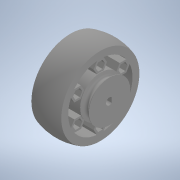
# Autodesk Inventor part: PulleyedWheelV1
Saved by Autodesk Inventor 2020 (Build 240168000, 168)
## iProperties
Created: 2023-12-21
Part Number: PulleyedWheelV1
Material: H TPU
Document SubType Name: Modeling
Designer: smz3rm
Density: 0.941117 g/cm^3
Appearance: Generic(1)
Mass: 15.4357 g
Surface Area: 101.181 cm^2
Volume: 16.4015 cm^3
d0: 3.000 mm
d1: 1.000 mm
d3: 34.000 mm
d4: 3.000 mm
d6: 18.000 mm
d7: 4.000 mm
d8: 0.00 deg
d9: 34.000 mm
d10: 1.600 mm
d11: 0.800 mm
d12: 6.000 ul
d16: 13.000 mm
d17: 0.00 deg
d20: 2.000 mm
d24: 1.000 mm
d26: 45.00 deg
Roundedness: 1.000 mm
d14: 360.00 deg
BaseThickness: 3.000 mm
TopThickness: 1.778 mm
SideThickness: 6.000 mm
BodyWidth: 130.000 mm
BodyLength: 150.000 mm
BodyHeight: 35.000 mm
DriveMotorHeight: 17.500 mm
WheelDia: 36.000 mm
WheelWidth: 13.000 mm
WheelGrooveWidth: 4.000 mm
WheelGrooveDia: 18.000 mm
WheelSlotWidth: 20.000 mm
WheelPulleyDia: 2.000 mm
WheeGuardlSlotWidth: 20.000 mm
Author: smz3rm
Autodesk Inventor part; units mm, degrees
ref_plane "YZ Plane" through (0, 0, 0) normal (1, 0, 0) x (0, 1, 0)
ref_plane "XZ Plane" through (0, 0, 0) normal (0, 1, 0) x (-1, 0, 0)
ref_plane "XY Plane" through (0, 0, 0) normal (0, 0, 1) x (1, 0, 0)
sketch "Sketch1" plane through (0, 0, 0) normal (1, 0, 0) x (0, 1, 0)
  circle A0 centre (0, 0) radius 1.5
  line L0 (-23.45, 0) -> (23.45, 0) projected
  line L1 (1.118, -1) -> (-1.118, -1)
  circle A1 centre (0, 0) radius 9
  circle A2 centre (0, 0) radius 17
  circle A3 centre (0, 0) radius 14
  dimension "d0" = 3
  dimension "d1" = 1
  dimension "d3" = 34
  dimension "d4" = 3
  dimension "d6" = 18
  constraints: 4 centre point, 4 coincident, 2 end point, 2 point on circle, 1 horizontal
  measures "d0" diameter of A0
  measures "d1" distance between parallel lines of L0 L1
  measures "d3" diameter of A2
  measures "d4" radial gap between concentric circles of A2 A3
  measures "d6" diameter of A1
extrude "Extrusion1" add sketch "Sketch1" along normal blind 4 contours L1 A0 | A0 L0 A1 | L0 A1 A0
sketch "Sketch3" plane through (0, 0, 0) normal (0, 0, 1) x (1, 0, 0)
  line L0 (0, 9) -> (4, 9) projected
  line L1 (-0.8, 0) -> (4.8, 0) projected
  circle A0 centre (1.3858, 8) radius 1
  line L2 (0.4001, 7.8312) -> (0.2, 9)
  line L3 (0, 9) -> (4, 9) projected
  line L4 (0, 10) -> (4, 10) projected
  line L5 (0, 9) -> (4, 9) projected
  line L6 (3.8, 9) -> (2.0929, 7.2929)
  line L7 (3.8, 9) -> (3.8, 9)
  line L8 (3.8, 9) -> (4, 9)
  line L9 (4, -9) -> (4, 9) projected
  line L10 (4, 9) -> (4, 9)
  line L11 (0, -9) -> (0, 9) projected
  line L12 (0.2, 9) -> (0, 9)
  point P0 (0, 0)
  point P1 (1.3858, 9)
  point P2 (3.8, 9)
  dimension "d20" = 2
  dimension "d26" = 45
  dimension "d28" = 0.2
  constraints: 12 end point, 3 perpendicular, 3 tangent, 2 collinear, 2 point on circle, 2 point on line, 1 centre point, 1 vertical, 3 other
  measures "d20" diameter of A0
  measures "d26" angle of L0 L6
  measures "d28" distance of L0.end L6.start
revolve "Revolution1" cut sketch "Sketch3" angle 360 about axis through (-10, 0, 0) along (-1, 0, 0) contours L0 A0 L2 | L0 L6 A0 | A0
sketch "Sketch2" plane through (0, 0, 0) normal (-1, 0, 0) x (0, 0, 1)
  circle A0 centre (0, 0) radius 17
  circle A1 centre (0, 0) radius 15.4
  circle A2 centre (0, 0) radius 9 projected
  line L0 (-1, 1.118) -> (-1, -1.118) projected
  arc A3 (-1, -1.118) -> (-1, 1.118) centre (0, 0) ccw projected
  line L1 (1.8714, 15.2859) -> (3.7427, 12.0446)
  line L2 (3.7427, 12.0446) -> (1.8714, 8.8033)
  line L3 (1.8714, 8.8033) -> (-1.8714, 8.8033)
  line L4 (-1.8714, 8.8033) -> (-3.7427, 12.0446)
  line L5 (-3.7427, 12.0446) -> (-1.8714, 15.2859)
  line L6 (-1.8714, 15.2859) -> (1.8714, 15.2859)
  line L7 (0, -23.45) -> (0, 23.45) projected
  line L8 (-1.4095, 14.4859) -> (-2.819, 12.0446)
  line L9 (-2.819, 12.0446) -> (-1.4095, 9.6033)
  line L10 (-1.4095, 9.6033) -> (1.4095, 9.6033)
  line L11 (1.4095, 9.6033) -> (2.819, 12.0446)
  line L12 (2.819, 12.0446) -> (1.4095, 14.4859)
  line L13 (1.4095, 14.4859) -> (-1.4095, 14.4859)
  line L14 (-12.3023, 2.781) -> (-14.1736, 6.0223)
  line L15 (-8.5596, 2.781) -> (-12.3023, 2.781)
  line L16 (-6.6882, 6.0223) -> (-8.5596, 2.781)
  line L17 (-14.1736, 6.0223) -> (-12.3023, 9.2636)
  line L18 (-12.3023, 9.2636) -> (-8.5596, 9.2636)
  line L19 (-8.5596, 9.2636) -> (-6.6882, 6.0223)
  line L20 (-11.8404, 8.4636) -> (-13.2499, 6.0223)
  line L21 (-13.2499, 6.0223) -> (-11.8404, 3.581)
  line L22 (-11.8404, 3.581) -> (-9.0214, 3.581)
  line L23 (-9.0214, 3.581) -> (-7.612, 6.0223)
  line L24 (-7.612, 6.0223) -> (-9.0214, 8.4636)
  line L25 (-9.0214, 8.4636) -> (-11.8404, 8.4636)
  line L26 (-8.5596, -9.2636) -> (-12.3023, -9.2636)
  line L27 (-6.6882, -6.0223) -> (-8.5596, -9.2636)
  line L28 (-8.5596, -2.781) -> (-6.6882, -6.0223)
  line L29 (-12.3023, -9.2636) -> (-14.1736, -6.0223)
  line L30 (-14.1736, -6.0223) -> (-12.3023, -2.781)
  line L31 (-12.3023, -2.781) -> (-8.5596, -2.781)
  line L32 (-13.2499, -6.0223) -> (-11.8404, -8.4636)
  line L33 (-11.8404, -8.4636) -> (-9.0214, -8.4636)
  line L34 (-9.0214, -8.4636) -> (-7.612, -6.0223)
  line L35 (-7.612, -6.0223) -> (-9.0214, -3.581)
  line L36 (-9.0214, -3.581) -> (-11.8404, -3.581)
  line L37 (-11.8404, -3.581) -> (-13.2499, -6.0223)
  line L38 (3.7427, -12.0446) -> (1.8714, -15.2859)
  line L39 (1.8714, -8.8033) -> (3.7427, -12.0446)
  line L40 (-1.8714, -8.8033) -> (1.8714, -8.8033)
  line L41 (1.8714, -15.2859) -> (-1.8714, -15.2859)
  line L42 (-1.8714, -15.2859) -> (-3.7427, -12.0446)
  line L43 (-3.7427, -12.0446) -> (-1.8714, -8.8033)
  line L44 (-1.4095, -14.4859) -> (1.4095, -14.4859)
  line L45 (1.4095, -14.4859) -> (2.819, -12.0446)
  line L46 (2.819, -12.0446) -> (1.4095, -9.6033)
  line L47 (1.4095, -9.6033) -> (-1.4095, -9.6033)
  line L48 (-1.4095, -9.6033) -> (-2.819, -12.0446)
  line L49 (-2.819, -12.0446) -> (-1.4095, -14.4859)
  line L50 (12.3023, -2.781) -> (14.1736, -6.0223)
  line L51 (8.5596, -2.781) -> (12.3023, -2.781)
  line L52 (6.6882, -6.0223) -> (8.5596, -2.781)
  line L53 (14.1736, -6.0223) -> (12.3023, -9.2636)
  line L54 (12.3023, -9.2636) -> (8.5596, -9.2636)
  line L55 (8.5596, -9.2636) -> (6.6882, -6.0223)
  line L56 (11.8404, -8.4636) -> (13.2499, -6.0223)
  line L57 (13.2499, -6.0223) -> (11.8404, -3.581)
  line L58 (11.8404, -3.581) -> (9.0214, -3.581)
  line L59 (9.0214, -3.581) -> (7.612, -6.0223)
  line L60 (7.612, -6.0223) -> (9.0214, -8.4636)
  line L61 (9.0214, -8.4636) -> (11.8404, -8.4636)
  line L62 (8.5596, 9.2636) -> (12.3023, 9.2636)
  line L63 (6.6882, 6.0223) -> (8.5596, 9.2636)
  line L64 (8.5596, 2.781) -> (6.6882, 6.0223)
  line L65 (12.3023, 9.2636) -> (14.1736, 6.0223)
  line L66 (14.1736, 6.0223) -> (12.3023, 2.781)
  line L67 (12.3023, 2.781) -> (8.5596, 2.781)
  line L68 (13.2499, 6.0223) -> (11.8404, 8.4636)
  line L69 (11.8404, 8.4636) -> (9.0214, 8.4636)
  line L70 (9.0214, 8.4636) -> (7.612, 6.0223)
  line L71 (7.612, 6.0223) -> (9.0214, 3.581)
  line L72 (9.0214, 3.581) -> (11.8404, 3.581)
  line L73 (11.8404, 3.581) -> (13.2499, 6.0223)
  point P0 (0, 12.0446)
  point P1 (-1.8714, -15.2859)
  point P2 (-12.3023, -9.2636)
  point P3 (-6.6882, -6.0223)
  point P4 (-1.8714, -8.8033)
  point P5 (-6.6882, 6.0223)
  point P6 (-12.3023, 9.2636)
  point P7 (12.3023, 9.2636)
  point P8 (6.6882, 6.0223)
  point P9 (1.8714, 8.8033)
  point P10 (14.1736, -6.0223)
  point P11 (8.5596, -2.781)
  point P12 (8.5596, 2.781)
  point P13 (14.1736, 6.0223)
  point P14 (1.8714, -15.2859)
  point P15 (1.8714, -8.8033)
  point P16 (12.3023, -9.2636)
  point P17 (-14.1736, 6.0223)
  point P18 (-8.5596, 2.781)
  point P19 (-8.5596, -2.781)
  point P20 (-14.1736, -6.0223)
  dimension "d9" = 34
  dimension "d10" = 1.6
  dimension "d11" = 0.8
  dimension "d14" = 360
  constraints: 144 end point, 2 centre point, 2 coincident, 2 point on circle, 1 point on line, 165 other
  measures "d9" diameter of A0
  measures "d10" radial gap between concentric circles of A0 A1
  measures "d11" distance between parallel lines of L5 L8
extrude "Extrusion2" add sketch "Sketch2" along normal blind 13 contours A0 L7 A1 | L7 A1 A0 | L7 L6 A1 | A1 L6 L7 | L7 L41 A1 | A1 L41 L7 | L1 L2 A2 L7 L10 L11 L12 L13 L6 | L6 L7 L13 L8 L9 L10 A2 L4 L5 | L42 L43 A2 L7 L47 L48 L49 L44 L41 | L41 L7 L44 L45 L46 L47 A2 L39 L38 | L65 L66 L67 A2 L63 L62 | A1 L65 | L17 A1 | L18 L19 A2 L15 L14 L17 | L29 L30 L31 A2 L27 L26 | A1 L29 | L53 A1 | L54 L55 A2 L51 L50 L53 | L3 L7 A2 | A2 L64 L52 L40 L7 A3 L3 | L3 L7 A3 L0 L40 A2 L28 L16 | A2 L7 L3 | L40 L7 A2 | A2 L7 L40 | A2 L64 | L16 A2 | A2 L28 | L52 A2
sketch "Sketch4" plane through (0, 0, 0) normal (0, 0, 1) x (1, 0, 0)
  line L0 (0, 17) -> (-13, 17) projected
  line L1 (-13, 17) -> (-13, -17) projected
  arc A0 (0, 17) -> (-13, 17) centre (-6.5, -3.625) ccw
  line L2 (-15.6, 0) -> (2.6, 0) projected
  point P0 (0, 0)
  point P1 (-6.5, 18)
  dimension "d24" = 1
  constraints: 3 point on circle, 1 centre point
  measures "d24" distance from line of L0 point (-6.5, 18)
revolve "Revolution2" add sketch "Sketch4" angle 360 about axis through (-10, 0, 0) along (1, 0, 0)
equation "\"d6\" = WheelGrooveDia"
equation "\"d7\" = WheelGrooveWidth"
equation "\"d20\" = WheelPulleyDia"
equation "\"d9\" = WheelDia - 2 * Roundedness"
equation "\"d16\" = WheelWidth"
equation "\"d24\" = Roundedness"
equation "\"Roundedness\" = 1"
equation "\"WheelGrooveDia\" = 18"
equation "\"WheelGrooveWidth\" = 4"
equation "\"WheelPulleyDia\" = 2"
equation "\"WheelDia\" = 36"
equation "\"WheelWidth\" = 13"
body "Solid1"
